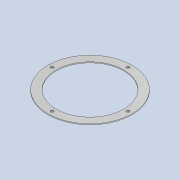
# Autodesk Inventor part: LightPoint_LedStripMetal
Saved by Autodesk Inventor 2020.3 (Build 243373010, 373A)
## iProperties
Created: 2020-12-04
Part Number: LightPoint_LedStripMetal
Material: Generic
Document SubType Name: Modeling
Designer: Yusuf
Mass: 2.34202 g
Surface Area: 52.5258 cm^2
Volume: 2.34202 cm^3
Density: 1 g/cm^3
Appearance: Default
Author: Yusuf
Autodesk Inventor part; units mm, degrees
ref_plane "YZ Plane" through (0, 0, 0) normal (1, 0, 0) x (0, 1, 0)
ref_plane "XZ Plane" through (0, 0, 0) normal (0, 1, 0) x (-1, 0, 0)
ref_plane "XY Plane" through (0, 0, 0) normal (0, 0, 1) x (1, 0, 0)
sketch "Sketch2" plane through (0, 0, 0) normal (0, 1, 0) x (-1, 0, 0)
  circle A0 centre (0, 0) radius 37.5
  circle A1 centre (0, 0) radius 46.5
  dimension "d14" = 75
  dimension "d15" = 9
  constraints: 2 centre point, 2 coincident
  measures "d14" diameter of A0
  measures "d15" radial gap between concentric circles of A1 A0
extrude "Extrusion1" add sketch "Sketch2" along normal blind 1
sketch "Sketch3" plane through (0, 1, 0) normal (0, 1, 0) x (1, 0, 0)
  circle A0 centre (0, 0) radius 46.5 projected
  line L0 (-46.5, 0) -> (-37.5, 0)
  circle A1 centre (0, 0) radius 37.5 projected
  circle A2 centre (0, 0) radius 42
  point P0 (-42, 0)
  point P1 (42, 0)
  point P2 (0, 42)
  point P3 (0, -42)
  constraints: 4 point on circle, 2 end point, 2 horizontal alignment, 1 centre point, 1 coincident, 1 horizontal, 1 midpoint, 2 other
hole "Hole1" at (-42, 1, 0) at (42, 1, 0) at (0, 1, -42) at (0, 1, 42) direction (0, -1, 0) diameter 3.242 depth 11.8 thread size "M4x0.7" class "6H" standard "ANSI Metric M Profile"
body "Solid1"
